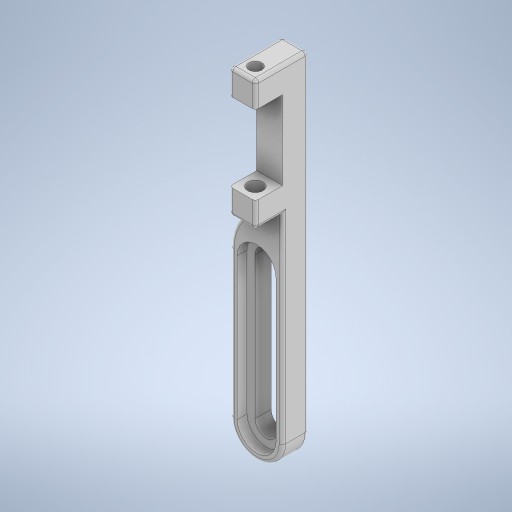
# Autodesk Inventor part: wiperholder
Saved by Autodesk Inventor 2024.2 (Build 282272000, 272)
## iProperties
Created: 2024-07-30
Part Number: wiperholder
Material: Generic
Document SubType Name: Modeling
Designer: Eric
Density: 1 g/cm^3
Appearance: Default
Author: Eric
Autodesk Inventor part; units mm, degrees
ref_plane "YZ Plane" through (0, 0, 0) normal (1, 0, 0) x (0, 1, 0)
ref_plane "XZ Plane" through (0, 0, 0) normal (0, 1, 0) x (-1, 0, 0)
ref_plane "XY Plane" through (0, 0, 0) normal (0, 0, 1) x (1, 0, 0)
ref_plane "Work Plane1" through (0, 0, 0) normal (0, 0, 1) x (1, 0, 0)
sketch "Sketch1" plane through (0, 0, 0) normal (0, 0, 1) x (1, 0, 0)
  circle A0 centre (-4, 62) radius 1.75 projected
  circle A1 centre (-4, 50) radius 1.75 projected
  line L0 (-8, 12) -> (-8, 66) projected
  line L1 (0, 66) -> (-8, 66) projected
  line L2 (0, 66) -> (0, 36)
  line L3 (0, 36) -> (-8, 36)
  line L4 (0, 66) -> (0, 91)
  line L5 (0, 91) -> (-4, 91)
  line L6 (-4, 91) -> (-4, 70)
  line L7 (-4, 70) -> (-8, 66)
  line L8 (-8, 66) -> (-8, 36)
  line L9 (-4, 62) -> (-4, 40) construction
  line L10 (-5.75, 62) -> (-5.75, 40)
  line L11 (-2.25, 40) -> (-2.25, 62)
  arc A2 (-2.25, 62) -> (-5.75, 62) centre (-4, 62) ccw
  arc A3 (-5.75, 40) -> (-2.25, 40) centre (-4, 40) ccw
  line L12 (-4, 80.5) -> (0, 80.5) construction
  point P0 (0, 0)
  point P1 (-4, 51)
  point P2 (-2.25, 62)
  dimension "d4" = 21
  dimension "d6" = 4
  dimension "d7" = 135
  dimension "d8" = 30
  dimension "d11" = 4
  dimension "d12" = 22
  dimension "d13" = 1.75
  constraints: 24 end point, 4 perpendicular, 4 point on circle, 4 tangent, 3 vertical, 2 centre point, 2 midpoint, 2 point on line, 1 collinear, 1 parallel
  measures "d4" distance from line of L6.end L5
  measures "d6" distance between parallel lines of L4 L6
  measures "d7" angle of L8 L7
  measures "d8" distance of L7.end L3.end
  measures "d11" horizontal distance of L9.start L7.end
  measures "d12" distance of L9.start L9.end
  measures "d13" radius of A3
extrude "Extrusion1" add sketch "Sketch1" along normal blind 4
sketch "Sketch2" plane through (0, 0, 4) normal (0, 0, 1) x (1, 0, 0)
  arc A0 (-2.25, 62) -> (-5.75, 62) centre (-4, 62) ccw projected
  arc A1 (-5.75, 40) -> (-2.25, 40) centre (-4, 40) ccw projected
  line L0 (-4, 62) -> (-4, 40) construction
  line L1 (-7, 62) -> (-7, 40)
  line L2 (-1, 40) -> (-1, 62)
  arc A2 (-1, 62) -> (-7, 62) centre (-4, 62) ccw
  arc A3 (-7, 40) -> (-1, 40) centre (-4, 40) ccw
  point P0 (0, 0)
  point P1 (-4, 51)
  dimension "d16" = 6
  constraints: 8 end point, 4 point on circle, 4 tangent, 2 centre point, 1 midpoint, 1 parallel, 1 vertical
  measures "d16" diameter of A3
extrude "Extrusion2" cut sketch "Sketch2" against normal blind 1.5
sketch "Sketch3" plane through (0, 0, 4) normal (0, 0, 1) x (1, 0, 0)
  line L0 (0, 36) -> (0, 91) projected
  line L1 (0, 87.1) -> (-4, 87.1)
  line L2 (-4, 91) -> (-4, 70) projected
  line L3 (-4, 71) -> (0, 71)
  line L4 (0, 74.9) -> (-4, 74.9)
  line L5 (0, 91) -> (-4, 91) projected
  point P0 (0, 0)
  point P1 (0, 70)
  dimension "d19" = 3.9
  dimension "d20" = 3.9
  dimension "d30" = 1
  constraints: 6 end point, 6 point on line, 2 horizontal, 2 perpendicular
  measures "d19" distance between parallel lines of L3 L4
  measures "d20" distance between parallel lines of L5 L1
  measures "d30" distance from line of L2.end L3
extrude "Extrusion3" add sketch "Sketch3" along normal blind 4.2 contours L3 L2 L4 L0 | L1 L2 L5 L0
sketch "Sketch4" plane through (-4, 91, 0) normal (0, 1, 0) x (1, 0, 0)
  circle A0 centre (2, -6.2) radius 1
  line L0 (4, -8.2) -> (0, -8.2) projected
  point P0 (4, 0)
  point P1 (2, -8.2)
  dimension "d23" = 2
  dimension "d24" = 2
  constraints: 1 centre point, 1 midpoint, 1 vertical alignment
  measures "d23" diameter of A0
  measures "d24" distance from line of L0 A0.centre
extrude "Extrusion4" cut sketch "Sketch4" against normal up to surface (3.9 mm away)
sketch "Sketch5" plane through (-4, 71, 4) normal (0, -1, 0) x (1, 0, 0)
  circle A0 centre (2, 2.2) radius 1 projected
  circle A1 centre (2, 2.2) radius 1.2
  point P0 (4, -4)
  dimension "d27" = 2.4
  constraints: 1 centre point, 1 coincident
  measures "d27" diameter of A1
extrude "Extrusion5" cut sketch "Sketch5" against normal up to surface (3.9 mm away) contours A0 | A1
fillet "Fillet1" radius 2.4 1 edges at (-4, 70, 2)
fillet "Fillet2" radius 4 2 edges at (-8, 36, 2) (0, 36, 2)
fillet "Fillet3" radius 8 1 edges at (-8, 66, 2)
fillet "Fillet4" radius 0.5 29 edges at (0, 91, 4.1) (-4, 91, 4.1) (-2, 91, 0) (-6.8285, 37.1715, 0) (-4, 36, 0) (-1.1715, 37.1715, 0) (-8, 51.3431, 0) (-7.391, 65.7478, 0) (-5.1799, 68.8201, 0) (-4.1827, 70.0757, 0) (-4, 80.9971, 0) (0, 65.5, 0) (-4, 89.05, 8.2) (-2, 91, 8.2) (0, 89.05, 8.2) (-4, 71, 6.1) (0, 71, 6.1) (-2, 71, 8.2) (-4, 72.95, 8.2) (0, 72.95, 8.2) (-5.1799, 68.8201, 4) (-4.1827, 70.0757, 4) (-4, 70.9971, 4) (-8, 51.3431, 4) (-6.8285, 37.1715, 4) (-4, 36, 4) (-1.1715, 37.1715, 4) (0, 55.4999, 4) (-7.391, 65.7478, 4)
body "Solid1"
